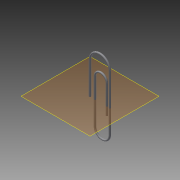
# Autodesk Inventor part: Paperclip
Saved by Autodesk Inventor 2015 (Build 190159000, 159)
## iProperties
Created: 2017-12-14
Part Number: Paperclip
Material: Generic
Document SubType Name: Modeling
Designer: Administrator
Density: 1 g/cm^3
Appearance: Default
Author: Administrator
Autodesk Inventor part; units mm, degrees
ref_plane "YZ Plane" through (0, 0, 0) normal (1, 0, 0) x (0, 1, 0)
ref_plane "XZ Plane" through (0, 0, 0) normal (0, 1, 0) x (-1, 0, 0)
ref_plane "XY Plane" through (0, 0, 0) normal (0, 0, 1) x (1, 0, 0)
sketch "Sketch1" plane through (0, 0, 0) normal (0, 0, 1) x (1, 0, 0)
  line L0 (0, 0) -> (0, 10.1643)
  line L1 (6.35, 10.1643) -> (6.35, -7.497)
  arc A0 (1.5875, -7.497) -> (6.35, -7.497) centre (3.9688, -7.497) ccw
  line L2 (1.5875, -7.497) -> (1.5875, 6.3755)
  arc A1 (5.3753, 6.35) -> (1.5875, 6.3755) centre (3.4815, 6.3755) ccw
  line L3 (5.3753, 6.35) -> (5.3753, -2.6068)
  arc A2 (6.35, 10.1643) -> (0, 10.1643) centre (3.175, 10.1643) ccw
  constraints: 8 end point, 6 point on circle, 4 tangent, 3 centre point, 3 vertical
ref_plane "Work Plane1" through (0, 0, 0) normal (0, 1, 0) x (-1, 0, 0)
sketch "Sketch2" plane through (0, 0, 0) normal (0, 1, 0) x (-1, 0, 0)
  circle A0 centre (0, 0) radius 0.2829
  constraints: 2 coincident, 1 centre point
sweep "Sweep1" add profiles "Sketch2" path "Sketch1"
body "Solid1"
